Autodesk Fusion 360 part; units mm, degrees
(part 3 of 4)
  arc A160 (-35.8833, 38.7193) -> (-35.3833, 38.2193) centre (-35.3833, 38.7193) ccw
  line L159 (-35.8833, 38.7193) -> (-35.8833, 51.7193)
  arc A161 (-16.8333, -104.1557) -> (-16.3333, -104.6557) centre (-16.3333, -104.1557) ccw
  line L160 (-16.8333, -104.1557) -> (-16.8333, -91.1557)
  arc A162 (-16.3333, -90.6557) -> (-16.8333, -91.1557) centre (-16.3333, -91.1557) ccw
  line L161 (-16.3333, -90.6557) -> (-3.3333, -90.6557)
  arc A163 (-2.8333, -91.1557) -> (-3.3333, -90.6557) centre (-3.3333, -91.1557) ccw
  line L162 (-2.8333, -91.1557) -> (-2.8333, -104.1557)
  arc A164 (-3.3333, -104.6557) -> (-2.8333, -104.1557) centre (-3.3333, -104.1557) ccw
  line L163 (-3.3333, -104.6557) -> (-16.3333, -104.6557)
  line L164 (35.2668, 213.6443) -> (35.2667, 200.6443)
  arc A165 (34.7667, 200.1443) -> (35.2667, 200.6443) centre (34.7667, 200.6443) ccw
  line L165 (34.7667, 200.1443) -> (21.7667, 200.1443)
  arc A166 (21.2668, 200.6443) -> (21.7667, 200.1443) centre (21.7667, 200.6443) ccw
  line L166 (21.2668, 200.6443) -> (21.2667, 213.6443)
  arc A167 (21.7667, 214.1443) -> (21.2667, 213.6443) centre (21.7668, 213.6443) ccw
  line L167 (21.7667, 214.1443) -> (34.7667, 214.1443)
  arc A168 (35.2668, 213.6443) -> (34.7667, 214.1443) centre (34.7667, 213.6443) ccw
  arc A169 (-41.4333, -78.462) -> (-40.9333, -77.962) centre (-41.4333, -77.962) ccw
  line L168 (-41.4333, -78.462) -> (-54.4333, -78.462)
  arc A170 (-54.9333, -77.962) -> (-54.4333, -78.462) centre (-54.4333, -77.962) ccw
  line L169 (-54.9333, -77.962) -> (-54.9333, -64.962)
  arc A171 (-54.4333, -64.462) -> (-54.9333, -64.962) centre (-54.4333, -64.962) ccw
  line L170 (-54.4333, -64.462) -> (-41.4333, -64.462)
  arc A172 (-40.9333, -64.962) -> (-41.4333, -64.462) centre (-41.4333, -64.962) ccw
  line L171 (-40.9333, -64.962) -> (-40.9333, -77.962)
  line L172 (58.5792, -47.5057) -> (45.5792, -47.5057)
  arc A173 (45.0792, -47.0057) -> (45.5792, -47.5057) centre (45.5792, -47.0057) ccw
  line L173 (45.0792, -47.0057) -> (45.0792, -34.0057)
  arc A174 (45.5792, -33.5057) -> (45.0792, -34.0057) centre (45.5792, -34.0057) ccw
  line L174 (45.5792, -33.5057) -> (58.5792, -33.5057)
  arc A175 (59.0792, -34.0057) -> (58.5792, -33.5057) centre (58.5793, -34.0057) ccw
  line L175 (59.0792, -34.0057) -> (59.0793, -47.0057)
  arc A176 (58.5792, -47.5057) -> (59.0793, -47.0057) centre (58.5792, -47.0057) ccw
  line L176 (35.2667, -100.6807) -> (35.2667, -113.6807)
  arc A177 (34.7667, -114.1807) -> (35.2667, -113.6807) centre (34.7667, -113.6807) ccw
  line L177 (34.7667, -114.1807) -> (21.7667, -114.1807)
  arc A178 (21.2667, -113.6807) -> (21.7667, -114.1807) centre (21.7667, -113.6807) ccw
  line L178 (21.2667, -113.6807) -> (21.2667, -100.6807)
  arc A179 (21.7667, -100.1807) -> (21.2667, -100.6807) centre (21.7667, -100.6807) ccw
  line L179 (21.7667, -100.1807) -> (34.7667, -100.1807)
  arc A180 (35.2667, -100.6807) -> (34.7667, -100.1807) centre (34.7667, -100.6807) ccw
  line L180 (-41.4333, -126.087) -> (-54.4333, -126.087)
  arc A181 (-54.9333, -125.587) -> (-54.4333, -126.087) centre (-54.4333, -125.587) ccw
  line L181 (-54.9333, -125.587) -> (-54.9333, -112.587)
  arc A182 (-54.4333, -112.087) -> (-54.9333, -112.587) centre (-54.4333, -112.587) ccw
  line L182 (-54.4333, -112.087) -> (-41.4333, -112.087)
  arc A183 (-40.9333, -112.587) -> (-41.4333, -112.087) centre (-41.4333, -112.587) ccw
  line L183 (-40.9333, -112.587) -> (-40.9332, -125.587)
  arc A184 (-41.4333, -126.087) -> (-40.9332, -125.587) centre (-41.4333, -125.587) ccw
  line L184 (45.5792, -114.4682) -> (58.5792, -114.4682)
  arc A185 (59.0792, -114.9682) -> (58.5792, -114.4682) centre (58.5792, -114.9682) ccw
  line L185 (59.0792, -114.9682) -> (59.0792, -127.9682)
  arc A186 (58.5792, -128.4682) -> (59.0792, -127.9682) centre (58.5792, -127.9682) ccw
  line L186 (58.5792, -128.4682) -> (45.5792, -128.4682)
  arc A187 (45.0792, -127.9682) -> (45.5792, -128.4682) centre (45.5792, -127.9682) ccw
  line L187 (45.0792, -127.9682) -> (45.0792, -114.9682)
  arc A188 (45.5792, -114.4682) -> (45.0792, -114.9682) centre (45.5792, -114.9682) ccw
  arc A189 (15.7167, 33.4568) -> (16.2167, 33.9568) centre (15.7167, 33.9568) ccw
  line L188 (15.7167, 33.4568) -> (2.7167, 33.4568)
  arc A190 (2.2167, 33.9568) -> (2.7167, 33.4568) centre (2.7167, 33.9568) ccw
  line L189 (2.2167, 33.9568) -> (2.2167, 46.9568)
  arc A191 (2.7167, 47.4568) -> (2.2167, 46.9568) centre (2.7167, 46.9568) ccw
  line L190 (2.7167, 47.4568) -> (15.7167, 47.4568)
  arc A192 (16.2167, 46.9568) -> (15.7167, 47.4568) centre (15.7167, 46.9568) ccw
  line L191 (16.2167, 46.9568) -> (16.2167, 33.9568)
  arc A193 (-44.9083, 156.9943) -> (-45.4083, 156.4943) centre (-44.9082, 156.4943) ccw
  line L192 (-44.9083, 156.9943) -> (-31.9083, 156.9943)
  arc A194 (-31.4083, 156.4943) -> (-31.9083, 156.9943) centre (-31.9083, 156.4943) ccw
  line L193 (-31.4083, 156.4943) -> (-31.4083, 143.4943)
  arc A195 (-31.9083, 142.9943) -> (-31.4083, 143.4943) centre (-31.9083, 143.4943) ccw
  line L194 (-31.9083, 142.9943) -> (-44.9083, 142.9943)
  arc A196 (-45.4083, 143.4943) -> (-44.9083, 142.9943) centre (-44.9083, 143.4943) ccw
  line L195 (-45.4083, 143.4943) -> (-45.4083, 156.4943)
  arc A197 (45.0792, 91.1068) -> (45.5793, 90.6068) centre (45.5792, 91.1068) ccw
  line L196 (45.0792, 91.1068) -> (45.0792, 104.1068)
  arc A198 (45.5792, 104.6068) -> (45.0792, 104.1068) centre (45.5792, 104.1068) ccw
  line L197 (45.5792, 104.6068) -> (58.5792, 104.6068)
  arc A199 (59.0792, 104.1068) -> (58.5792, 104.6068) centre (58.5792, 104.1068) ccw
  line L198 (59.0792, 104.1068) -> (59.0792, 91.1068)
  arc A200 (58.5793, 90.6068) -> (59.0792, 91.1068) centre (58.5792, 91.1068) ccw
  line L199 (58.5793, 90.6068) -> (45.5793, 90.6068)
  line L200 (-46.8463, 155.4943) -> (-46.8463, 141.4943)
  arc A201 (-47.3463, 140.9943) -> (-46.8463, 141.4943) centre (-47.3463, 141.4943) ccw
  line L201 (-47.3463, 140.9943) -> (-53.3463, 140.9943)
  arc A202 (-53.8463, 141.4943) -> (-53.3463, 140.9943) centre (-53.3463, 141.4943) ccw
  line L202 (-53.8463, 141.4943) -> (-53.8462, 155.4943)
  arc A203 (-53.3463, 155.9943) -> (-53.8462, 155.4943) centre (-53.3463, 155.4943) ccw
  line L203 (-53.3463, 155.9943) -> (-47.3463, 155.9943)
  arc A204 (-46.8463, 155.4943) -> (-47.3463, 155.9943) centre (-47.3463, 155.4943) ccw
  line L204 (34.7667, 57.2693) -> (21.7667, 57.2693)
  arc A205 (21.2667, 57.7693) -> (21.7667, 57.2693) centre (21.7667, 57.7693) ccw
  line L205 (21.2667, 57.7693) -> (21.2667, 70.7693)
  arc A206 (21.7667, 71.2693) -> (21.2667, 70.7693) centre (21.7667, 70.7693) ccw
  line L206 (21.7667, 71.2693) -> (34.7667, 71.2693)
  arc A207 (35.2667, 70.7693) -> (34.7667, 71.2693) centre (34.7667, 70.7693) ccw
  line L207 (35.2667, 70.7693) -> (35.2667, 57.7693)
  arc A208 (34.7667, 57.2693) -> (35.2667, 57.7693) centre (34.7667, 57.7693) ccw
  line L208 (16.2167, -29.2432) -> (16.2167, -42.2432)
  arc A209 (15.7167, -42.7432) -> (16.2167, -42.2432) centre (15.7167, -42.2432) ccw
  line L209 (15.7167, -42.7432) -> (2.7167, -42.7432)
  arc A210 (2.2167, -42.2432) -> (2.7167, -42.7432) centre (2.7167, -42.2432) ccw
  line L210 (2.2167, -42.2432) -> (2.2167, -29.2432)
  arc A211 (2.7167, -28.7432) -> (2.2167, -29.2432) centre (2.7167, -29.2432) ccw
  line L211 (2.7167, -28.7432) -> (15.7167, -28.7432)
  arc A212 (16.2167, -29.2432) -> (15.7167, -28.7432) centre (15.7167, -29.2432) ccw
  line L212 (67.9431, 166.6443) -> (37.7667, 166.6443)
  line L213 (37.7667, 166.6443) -> (37.7668, 228.6)
  line L214 (37.7668, 228.6) -> (-61.7708, 228.6)
  line L215 (-61.7708, 228.6) -> (-61.7708, -231.4)
  line L216 (-61.7708, -231.4) -> (63.3431, -231.4)
  line L217 (63.3431, -231.4) -> (67.9431, -231.4)
  line L218 (67.9431, -231.4) -> (67.9431, 166.6443)
  line L219 (-2.8333, -53.0557) -> (-2.8333, -66.0557)
  arc A213 (-3.3333, -66.5557) -> (-2.8333, -66.0557) centre (-3.3333, -66.0557) ccw
  line L220 (-3.3333, -66.5557) -> (-16.3333, -66.5557)
  arc A214 (-16.8333, -66.0557) -> (-16.3333, -66.5557) centre (-16.3333, -66.0557) ccw
  line L221 (-16.8333, -66.0557) -> (-16.8333, -53.0557)
  arc A215 (-16.3333, -52.5557) -> (-16.8333, -53.0557) centre (-16.3333, -53.0557) ccw
  line L222 (-16.3333, -52.5557) -> (-3.3333, -52.5557)
  arc A216 (-2.8333, -53.0557) -> (-3.3333, -52.5557) centre (-3.3333, -53.0557) ccw
  line L223 (-37.8833, 120.8323) -> (-37.8833, 126.8323)
  arc A217 (-37.3833, 127.3323) -> (-37.8833, 126.8323) centre (-37.3833, 126.8323) ccw
  line L224 (-37.3833, 127.3323) -> (-23.3833, 127.3323)
  arc A218 (-22.8833, 126.8323) -> (-23.3833, 127.3323) centre (-23.3833, 126.8323) ccw
  line L225 (-22.8833, 126.8323) -> (-22.8833, 120.8323)
  arc A219 (-23.3833, 120.3323) -> (-22.8833, 120.8323) centre (-23.3833, 120.8323) ccw
  line L226 (-23.3833, 120.3323) -> (-37.3833, 120.3323)
  arc A220 (-37.8833, 120.8323) -> (-37.3833, 120.3323) centre (-37.3833, 120.8323) ccw
  arc A221 (2.7167, 85.5568) -> (2.2167, 85.0568) centre (2.7167, 85.0568) ccw
  line L227 (2.7167, 85.5568) -> (15.7167, 85.5568)
  arc A222 (16.2167, 85.0568) -> (15.7167, 85.5568) centre (15.7167, 85.0568) ccw
  line L228 (16.2167, 85.0568) -> (16.2167, 72.0568)
  arc A223 (15.7167, 71.5568) -> (16.2167, 72.0568) centre (15.7167, 72.0568) ccw
  line L229 (15.7167, 71.5568) -> (2.7167, 71.5568)
  arc A224 (2.2167, 72.0568) -> (2.7167, 71.5568) centre (2.7167, 72.0568) ccw
  line L230 (2.2167, 72.0568) -> (2.2167, 85.0568)
  arc A225 (15.7167, 162.0443) -> (16.2168, 162.5443) centre (15.7167, 162.5443) ccw
  line L231 (15.7167, 162.0443) -> (2.7168, 162.0443)
  arc A226 (2.2167, 162.5443) -> (2.7168, 162.0443) centre (2.7168, 162.5443) ccw
  line L232 (2.2167, 162.5443) -> (2.2168, 175.5443)
  arc A227 (2.7168, 176.0443) -> (2.2168, 175.5443) centre (2.7167, 175.5443) ccw
  line L233 (2.7168, 176.0443) -> (15.7167, 176.0443)
  arc A228 (16.2168, 175.5443) -> (15.7167, 176.0443) centre (15.7168, 175.5443) ccw
  line L234 (16.2168, 175.5443) -> (16.2168, 162.5443)
  line L235 (-22.9703, 155.4943) -> (-22.9703, 141.4943)
  arc A229 (-23.4703, 140.9943) -> (-22.9703, 141.4943) centre (-23.4703, 141.4943) ccw
  line L236 (-23.4703, 140.9943) -> (-29.4703, 140.9943)
  arc A230 (-29.9703, 141.4943) -> (-29.4703, 140.9943) centre (-29.4703, 141.4943) ccw
  line L237 (-29.9703, 141.4943) -> (-29.9703, 155.4943)
  arc A231 (-29.4703, 155.9943) -> (-29.9703, 155.4943) centre (-29.4702, 155.4943) ccw
  line L238 (-29.4703, 155.9943) -> (-23.4703, 155.9943)
  arc A232 (-22.9703, 155.4943) -> (-23.4703, 155.9943) centre (-23.4703, 155.4943) ccw
  line L239 (-16.3333, -33.5057) -> (-3.3333, -33.5057)
  arc A233 (-2.8333, -34.0057) -> (-3.3333, -33.5057) centre (-3.3333, -34.0057) ccw
  line L240 (-2.8333, -34.0057) -> (-2.8333, -47.0057)
  arc A234 (-3.3333, -47.5057) -> (-2.8333, -47.0057) centre (-3.3333, -47.0057) ccw
  line L241 (-3.3333, -47.5057) -> (-16.3333, -47.5057)
  arc A235 (-16.8333, -47.0057) -> (-16.3333, -47.5057) centre (-16.3333, -47.0057) ccw
  line L242 (-16.8333, -47.0057) -> (-16.8333, -34.0057)
  arc A236 (-16.3333, -33.5057) -> (-16.8333, -34.0057) centre (-16.3333, -34.0057) ccw
  line L243 (-21.8833, -181.6432) -> (-21.8833, -194.6432)
  arc A237 (-22.3833, -195.1432) -> (-21.8833, -194.6432) centre (-22.3833, -194.6432) ccw
  line L244 (-22.3833, -195.1432) -> (-35.3833, -195.1432)
  arc A238 (-35.8833, -194.6432) -> (-35.3833, -195.1432) centre (-35.3833, -194.6432) ccw
  line L245 (-35.8833, -194.6432) -> (-35.8833, -181.6432)
  arc A239 (-35.3833, -181.1432) -> (-35.8833, -181.6432) centre (-35.3833, -181.6432) ccw
  line L246 (-35.3833, -181.1432) -> (-22.3833, -181.1432)
  arc A240 (-21.8833, -181.6432) -> (-22.3833, -181.1432) centre (-22.3833, -181.6432) ccw
  arc A241 (2.7167, -9.6932) -> (2.2168, -10.1932) centre (2.7167, -10.1932) ccw
  line L247 (2.7167, -9.6932) -> (15.7167, -9.6932)
  arc A242 (16.2167, -10.1932) -> (15.7167, -9.6932) centre (15.7167, -10.1932) ccw
  line L248 (16.2167, -10.1932) -> (16.2167, -23.1932)
  arc A243 (15.7167, -23.6932) -> (16.2167, -23.1932) centre (15.7167, -23.1932) ccw
  line L249 (15.7167, -23.6932) -> (2.7167, -23.6932)
  arc A244 (2.2167, -23.1932) -> (2.7167, -23.6932) centre (2.7167, -23.1932) ccw
  line L250 (2.2167, -23.1932) -> (2.2168, -10.1932)
  line L251 (-54.9333, -101.7745) -> (-54.9333, -88.7745)
  arc A245 (-54.4333, -88.2745) -> (-54.9333, -88.7745) centre (-54.4333, -88.7745) ccw
  line L252 (-54.4333, -88.2745) -> (-41.4333, -88.2745)
  arc A246 (-40.9333, -88.7745) -> (-41.4333, -88.2745) centre (-41.4333, -88.7745) ccw
  line L253 (-40.9333, -88.7745) -> (-40.9333, -101.7745)
  arc A247 (-41.4333, -102.2745) -> (-40.9333, -101.7745) centre (-41.4333, -101.7745) ccw
  line L254 (-41.4333, -102.2745) -> (-54.4333, -102.2745)
  arc A248 (-54.9333, -101.7745) -> (-54.4333, -102.2745) centre (-54.4333, -101.7745) ccw
  circle A249 centre (42.9431, 161.6443) radius 1.5
  arc A250 (-21.8833, 32.6693) -> (-22.3833, 33.1693) centre (-22.3833, 32.6693) ccw
  line L255 (-21.8833, 32.6693) -> (-21.8833, 19.6693)
  arc A251 (-22.3833, 19.1693) -> (-21.8833, 19.6693) centre (-22.3833, 19.6693) ccw
  line L256 (-22.3833, 19.1693) -> (-35.3833, 19.1693)
  arc A252 (-35.8833, 19.6693) -> (-35.3833, 19.1693) centre (-35.3833, 19.6693) ccw
  line L257 (-35.8833, 19.6693) -> (-35.8833, 32.6693)
  arc A253 (-35.3833, 33.1693) -> (-35.8833, 32.6693) centre (-35.3833, 32.6693) ccw
  line L258 (-35.3833, 33.1693) -> (-22.3833, 33.1693)
  line L259 (35.2667, 32.6693) -> (35.2667, 19.6693)
  arc A254 (34.7667, 19.1693) -> (35.2667, 19.6693) centre (34.7667, 19.6693) ccw
  line L260 (34.7667, 19.1693) -> (21.7667, 19.1693)
  arc A255 (21.2667, 19.6693) -> (21.7667, 19.1693) centre (21.7667, 19.6693) ccw
  line L261 (21.2667, 19.6693) -> (21.2667, 32.6693)
  arc A256 (21.7667, 33.1693) -> (21.2667, 32.6693) centre (21.7667, 32.6693) ccw
  line L262 (21.7667, 33.1693) -> (34.7667, 33.1693)
  arc A257 (35.2667, 32.6693) -> (34.7667, 33.1693) centre (34.7667, 32.6693) ccw
  arc A258 (-2.8333, 123.1568) -> (-3.3333, 123.6568) centre (-3.3333, 123.1568) ccw
  line L263 (-2.8333, 123.1568) -> (-2.8333, 110.1568)
  arc A259 (-3.3333, 109.6568) -> (-2.8333, 110.1568) centre (-3.3333, 110.1568) ccw
  line L264 (-3.3333, 109.6568) -> (-16.3333, 109.6568)
  arc A260 (-16.8333, 110.1568) -> (-16.3333, 109.6568) centre (-16.3333, 110.1568) ccw
  line L265 (-16.8333, 110.1568) -> (-16.8333, 123.1568)
  arc A261 (-16.3333, 123.6568) -> (-16.8333, 123.1568) centre (-16.3333, 123.1568) ccw
  line L266 (-16.3333, 123.6568) -> (-3.3333, 123.6568)
  line L267 (35.2667, 89.8193) -> (35.2667, 76.8193)
  arc A262 (34.7667, 76.3193) -> (35.2667, 76.8193) centre (34.7667, 76.8193) ccw
  line L268 (34.7667, 76.3193) -> (21.7667, 76.3193)
  arc A263 (21.2667, 76.8193) -> (21.7667, 76.3193) centre (21.7667, 76.8193) ccw
  line L269 (21.2667, 76.8193) -> (21.2667, 89.8193)
  arc A264 (21.7667, 90.3193) -> (21.2667, 89.8193) centre (21.7667, 89.8193) ccw
  line L270 (21.7667, 90.3193) -> (34.7667, 90.3193)
  arc A265 (35.2667, 89.8193) -> (34.7667, 90.3193) centre (34.7667, 89.8193) ccw
  line L271 (-35.3833, -62.0807) -> (-22.3833, -62.0807)
  arc A266 (-21.8833, -62.5807) -> (-22.3833, -62.0807) centre (-22.3833, -62.5807) ccw
  line L272 (-21.8833, -62.5807) -> (-21.8833, -75.5807)
  arc A267 (-22.3833, -76.0807) -> (-21.8833, -75.5807) centre (-22.3833, -75.5807) ccw
  line L273 (-22.3833, -76.0807) -> (-35.3833, -76.0807)
  arc A268 (-35.8833, -75.5807) -> (-35.3833, -76.0807) centre (-35.3833, -75.5807) ccw
  line L274 (-35.8833, -75.5807) -> (-35.8833, -62.5807)
  arc A269 (-35.3833, -62.0807) -> (-35.8833, -62.5807) centre (-35.3833, -62.5807) ccw
  arc A270 (21.7667, -23.9807) -> (21.2667, -24.4807) centre (21.7667, -24.4807) ccw
  line L275 (21.7667, -23.9807) -> (34.7667, -23.9807)
  arc A271 (35.2667, -24.4807) -> (34.7667, -23.9807) centre (34.7667, -24.4807) ccw
  line L276 (35.2667, -24.4807) -> (35.2667, -37.4807)
  arc A272 (34.7667, -37.9807) -> (35.2667, -37.4807) centre (34.7667, -37.4807) ccw
  line L277 (34.7667, -37.9807) -> (21.7667, -37.9807)
  arc A273 (21.2667, -37.4807) -> (21.7667, -37.9807) centre (21.7667, -37.4807) ccw
  line L278 (21.2667, -37.4807) -> (21.2667, -24.4807)
  line L279 (-40.9333, -162.5932) -> (-40.9333, -175.5932)
  arc A274 (-41.4333, -176.0932) -> (-40.9333, -175.5932) centre (-41.4333, -175.5932) ccw
  line L280 (-41.4333, -176.0932) -> (-54.4333, -176.0932)
  arc A275 (-54.9333, -175.5932) -> (-54.4333, -176.0932) centre (-54.4333, -175.5932) ccw
  line L281 (-54.9333, -175.5932) -> (-54.9333, -162.5932)
  arc A276 (-54.4333, -162.0932) -> (-54.9333, -162.5932) centre (-54.4333, -162.5932) ccw
  line L282 (-54.4333, -162.0932) -> (-41.4333, -162.0932)
  arc A277 (-40.9333, -162.5932) -> (-41.4333, -162.0932) centre (-41.4333, -162.5932) ccw
  arc A278 (58.5792, -71.3182) -> (59.0793, -70.8182) centre (58.5792, -70.8182) ccw
  line L283 (58.5792, -71.3182) -> (45.5792, -71.3182)
  arc A279 (45.0792, -70.8182) -> (45.5792, -71.3182) centre (45.5792, -70.8182) ccw
  line L284 (45.0792, -70.8182) -> (45.0792, -57.8182)
  arc A280 (45.5792, -57.3182) -> (45.0792, -57.8182) centre (45.5792, -57.8182) ccw
  line L285 (45.5792, -57.3182) -> (58.5792, -57.3182)
  arc A281 (59.0792, -57.8182) -> (58.5792, -57.3182) centre (58.5792, -57.8182) ccw
  line L286 (59.0792, -57.8182) -> (59.0793, -70.8182)
  line L287 (16.2167, 194.5943) -> (16.2168, 181.5943)
  arc A282 (15.7167, 181.0943) -> (16.2168, 181.5943) centre (15.7167, 181.5943) ccw
  line L288 (15.7167, 181.0943) -> (2.7168, 181.0943)
  arc A283 (2.2168, 181.5943) -> (2.7168, 181.0943) centre (2.7167, 181.5943) ccw
  line L289 (2.2168, 181.5943) -> (2.2167, 194.5943)
  arc A284 (2.7168, 195.0943) -> (2.2167, 194.5943) centre (2.7167, 194.5943) ccw
  line L290 (2.7168, 195.0943) -> (15.7168, 195.0943)
  arc A285 (16.2167, 194.5943) -> (15.7168, 195.0943) centre (15.7167, 194.5943) ccw
  arc A286 (-35.8833, 105.3943) -> (-35.3833, 104.8943) centre (-35.3833, 105.3943) ccw
  line L291 (-35.8833, 105.3943) -> (-35.8833, 118.3943)
  arc A287 (-35.3833, 118.8943) -> (-35.8833, 118.3943) centre (-35.3833, 118.3943) ccw
  line L292 (-35.3833, 118.8943) -> (-22.3833, 118.8943)
  arc A288 (-21.8833, 118.3943) -> (-22.3833, 118.8943) centre (-22.3833, 118.3943) ccw
  line L293 (-21.8833, 118.3943) -> (-21.8833, 105.3943)
  arc A289 (-22.3833, 104.8943) -> (-21.8833, 105.3943) centre (-22.3833, 105.3943) ccw
  line L294 (-22.3833, 104.8943) -> (-35.3833, 104.8943)
  line L295 (-41.4333, 190.6193) -> (-54.4333, 190.6193)
  arc A290 (-54.9332, 191.1193) -> (-54.4333, 190.6193) centre (-54.4333, 191.1193) ccw
  line L296 (-54.9332, 191.1193) -> (-54.9332, 204.1193)
  arc A291 (-54.4332, 204.6193) -> (-54.9332, 204.1193) centre (-54.4333, 204.1193) ccw
  line L297 (-54.4332, 204.6193) -> (-41.4333, 204.6193)
  arc A292 (-40.9332, 204.1193) -> (-41.4333, 204.6193) centre (-41.4332, 204.1193) ccw
  line L298 (-40.9332, 204.1193) -> (-40.9333, 191.1193)
  arc A293 (-41.4333, 190.6193) -> (-40.9333, 191.1193) centre (-41.4333, 191.1193) ccw
  arc A294 (-16.8333, -85.1057) -> (-16.3333, -85.6057) centre (-16.3333, -85.1057) ccw
  line L299 (-16.8333, -85.1057) -> (-16.8333, -72.1057)
  arc A295 (-16.3333, -71.6057) -> (-16.8333, -72.1057) centre (-16.3333, -72.1057) ccw
  line L300 (-16.3333, -71.6057) -> (-3.3333, -71.6057)
  arc A296 (-2.8333, -72.1057) -> (-3.3333, -71.6057) centre (-3.3333, -72.1057) ccw
  line L301 (-2.8333, -72.1057) -> (-2.8333, -85.1057)
  arc A297 (-3.3333, -85.6057) -> (-2.8333, -85.1057) centre (-3.3333, -85.1057) ccw
  line L302 (-3.3333, -85.6057) -> (-16.3333, -85.6057)
  line L303 (-35.3833, 195.0943) -> (-22.3833, 195.0943)
  arc A298 (-21.8833, 194.5943) -> (-22.3833, 195.0943) centre (-22.3832, 194.5943) ccw
  line L304 (-21.8833, 194.5943) -> (-21.8833, 181.5943)
  arc A299 (-22.3833, 181.0943) -> (-21.8833, 181.5943) centre (-22.3833, 181.5943) ccw
  line L305 (-22.3833, 181.0943) -> (-35.3833, 181.0943)
  arc A300 (-35.8833, 181.5943) -> (-35.3833, 181.0943) centre (-35.3833, 181.5943) ccw
  line L306 (-35.8833, 181.5943) -> (-35.8833, 194.5943)
  arc A301 (-35.3833, 195.0943) -> (-35.8833, 194.5943) centre (-35.3833, 194.5943) ccw
  line L307 (15.7167, 14.4068) -> (2.7167, 14.4068)
  arc A302 (2.2167, 14.9068) -> (2.7167, 14.4068) centre (2.7167, 14.9068) ccw
  line L308 (2.2167, 14.9068) -> (2.2167, 27.9068)
  arc A303 (2.7167, 28.4068) -> (2.2167, 27.9068) centre (2.7167, 27.9068) ccw
  line L309 (2.7167, 28.4068) -> (15.7167, 28.4068)
  arc A304 (16.2167, 27.9068) -> (15.7167, 28.4068) centre (15.7167, 27.9068) ccw
  line L310 (16.2167, 27.9068) -> (16.2167, 14.9068)
  arc A305 (15.7167, 14.4068) -> (16.2167, 14.9068) centre (15.7167, 14.9068) ccw
  line L311 (-16.8333, 10.1443) -> (-16.8333, 23.1443)
  arc A306 (-16.3333, 23.6443) -> (-16.8333, 23.1443) centre (-16.3333, 23.1443) ccw
  line L312 (-16.3333, 23.6443) -> (-3.3333, 23.6443)
  arc A307 (-2.8333, 23.1443) -> (-3.3333, 23.6443) centre (-3.3333, 23.1443) ccw
  line L313 (-2.8333, 23.1443) -> (-2.8333, 10.1443)
  arc A308 (-3.3333, 9.6443) -> (-2.8333, 10.1443) centre (-3.3333, 10.1443) ccw
  line L314 (-3.3333, 9.6443) -> (-16.3333, 9.6443)
  arc A309 (-16.8333, 10.1443) -> (-16.3333, 9.6443) centre (-16.3333, 10.1443) ccw
  line L315 (25.2417, -195.1432) -> (12.2417, -195.1432)
  arc A310 (11.7417, -194.6432) -> (12.2417, -195.1432) centre (12.2417, -194.6432) ccw
  line L316 (11.7417, -194.6432) -> (11.7417, -181.6432)
  arc A311 (12.2417, -181.1432) -> (11.7417, -181.6432) centre (12.2417, -181.6432) ccw
  line L317 (12.2417, -181.1432) -> (25.2417, -181.1432)
  arc A312 (25.7417, -181.6432) -> (25.2417, -181.1432) centre (25.2417, -181.6432) ccw
  line L318 (25.7417, -181.6432) -> (25.7417, -194.6432)
  arc A313 (25.2417, -195.1432) -> (25.7417, -194.6432) centre (25.2417, -194.6432) ccw
  arc A314 (-40.9333, 125.538) -> (-41.4333, 126.038) centre (-41.4333, 125.538) ccw
  line L319 (-40.9333, 125.538) -> (-40.9333, 112.538)
  arc A315 (-41.4333, 112.038) -> (-40.9333, 112.538) centre (-41.4333, 112.538) ccw
  line L320 (-41.4333, 112.038) -> (-54.4333, 112.038)
  arc A316 (-54.9333, 112.538) -> (-54.4333, 112.038) centre (-54.4333, 112.538) ccw
  line L321 (-54.9333, 112.538) -> (-54.9333, 125.538)
  arc A317 (-54.4333, 126.038) -> (-54.9333, 125.538) centre (-54.4333, 125.538) ccw
  line L322 (-54.4333, 126.038) -> (-41.4333, 126.038)
  arc A318 (-37.3833, 103.4563) -> (-37.8833, 102.9563) centre (-37.3833, 102.9563) ccw
  line L323 (-37.3833, 103.4563) -> (-23.3833, 103.4563)
  arc A319 (-22.8833, 102.9563) -> (-23.3833, 103.4563) centre (-23.3833, 102.9563) ccw
  line L324 (-22.8833, 102.9563) -> (-22.8833, 96.9563)
  arc A320 (-23.3833, 96.4563) -> (-22.8833, 96.9563) centre (-23.3833, 96.9563) ccw
  line L325 (-23.3833, 96.4563) -> (-37.3833, 96.4563)
  arc A321 (-37.8833, 96.9563) -> (-37.3833, 96.4563) centre (-37.3833, 96.9563) ccw
  line L326 (-37.8833, 96.9563) -> (-37.8833, 102.9563)
  arc A322 (6.6917, -162.5932) -> (6.1917, -162.0932) centre (6.1917, -162.5932) ccw
  line L327 (6.6917, -162.5932) -> (6.6917, -175.5932)
  arc A323 (6.1917, -176.0932) -> (6.6917, -175.5932) centre (6.1917, -175.5932) ccw
  line L328 (6.1917, -176.0932) -> (-6.8083, -176.0932)
  arc A324 (-7.3083, -175.5932) -> (-6.8083, -176.0932) centre (-6.8083, -175.5932) ccw
  line L329 (-7.3083, -175.5932) -> (-7.3083, -162.5932)
  arc A325 (-6.8083, -162.0932) -> (-7.3083, -162.5932) centre (-6.8083, -162.5932) ccw
  line L330 (-6.8083, -162.0932) -> (6.1917, -162.0932)
  arc A326 (15.7167, -118.9432) -> (16.2167, -118.4432) centre (15.7167, -118.4432) ccw
  line L331 (15.7167, -118.9432) -> (2.7167, -118.9432)
  arc A327 (2.2167, -118.4432) -> (2.7167, -118.9432) centre (2.7167, -118.4432) ccw
  line L332 (2.2167, -118.4432) -> (2.2167, -105.4432)
  arc A328 (2.7167, -104.9432) -> (2.2167, -105.4432) centre (2.7167, -105.4432) ccw
  line L333 (2.7167, -104.9432) -> (15.7167, -104.9432)
  arc A329 (16.2167, -105.4432) -> (15.7167, -104.9432) centre (15.7167, -105.4432) ccw
  line L334 (16.2167, -105.4432) -> (16.2167, -118.4432)
  line L335 (-3.3333, 85.8443) -> (-16.3333, 85.8443)
  arc A330 (-16.8333, 86.3443) -> (-16.3333, 85.8443) centre (-16.3333, 86.3443) ccw
  line L336 (-16.8333, 86.3443) -> (-16.8333, 99.3443)
  arc A331 (-16.3333, 99.8443) -> (-16.8333, 99.3443) centre (-16.3333, 99.3443) ccw
  line L337 (-16.3333, 99.8443) -> (-3.3333, 99.8443)
  arc A332 (-2.8333, 99.3443) -> (-3.3333, 99.8443) centre (-3.3333, 99.3443) ccw
  line L338 (-2.8333, 99.3443) -> (-2.8332, 86.3443)
  arc A333 (-3.3333, 85.8443) -> (-2.8332, 86.3443) centre (-3.3333, 86.3443) ccw
  line L339 (-3.3333, 47.7443) -> (-16.3333, 47.7443)
  arc A334 (-16.8333, 48.2443) -> (-16.3333, 47.7443) centre (-16.3333, 48.2443) ccw
  line L340 (-16.8333, 48.2443) -> (-16.8333, 61.2443)
  arc A335 (-16.3333, 61.7443) -> (-16.8333, 61.2443) centre (-16.3333, 61.2443) ccw
  line L341 (-16.3333, 61.7443) -> (-3.3333, 61.7443)
  arc A336 (-2.8333, 61.2443) -> (-3.3333, 61.7443) centre (-3.3333, 61.2443) ccw
  line L342 (-2.8333, 61.2443) -> (-2.8333, 48.2443)
  arc A337 (-3.3333, 47.7443) -> (-2.8333, 48.2443) centre (-3.3333, 48.2443) ccw
  line L343 (35.2667, -127.3495) -> (35.2667, -140.3495)
  arc A338 (34.7667, -140.8495) -> (35.2667, -140.3495) centre (34.7667, -140.3495) ccw
  line L344 (34.7667, -140.8495) -> (21.7667, -140.8495)
  arc A339 (21.2667, -140.3495) -> (21.7667, -140.8495) centre (21.7667, -140.3495) ccw
  line L345 (21.2667, -140.3495) -> (21.2667, -127.3495)
  arc A340 (21.7667, -126.8495) -> (21.2667, -127.3495) centre (21.7667, -127.3495) ccw
  line L346 (21.7667, -126.8495) -> (34.7667, -126.8495)
  arc A341 (35.2667, -127.3495) -> (34.7667, -126.8495) centre (34.7667, -127.3495) ccw
  arc A342 (58.5792, -109.4182) -> (59.0792, -108.9182) centre (58.5792, -108.9182) ccw
  line L347 (58.5792, -109.4182) -> (45.5792, -109.4182)
  arc A343 (45.0792, -108.9182) -> (45.5792, -109.4182) centre (45.5792, -108.9182) ccw
  line L348 (45.0792, -108.9182) -> (45.0792, -95.9182)
  arc A344 (45.5792, -95.4182) -> (45.0792, -95.9182) centre (45.5792, -95.9182) ccw
  line L349 (45.5792, -95.4182) -> (58.5792, -95.4182)
  arc A345 (59.0792, -95.9182) -> (58.5792, -95.4182) centre (58.5792, -95.9182) ccw
  line L350 (59.0792, -95.9182) -> (59.0792, -108.9182)
  line L351 (-35.3833, -81.1307) -> (-22.3833, -81.1307)
  arc A346 (-21.8833, -81.6307) -> (-22.3833, -81.1307) centre (-22.3833, -81.6307) ccw
  line L352 (-21.8833, -81.6307) -> (-21.8833, -94.6307)
  arc A347 (-22.3833, -95.1307) -> (-21.8833, -94.6307) centre (-22.3833, -94.6307) ccw
  line L353 (-22.3833, -95.1307) -> (-35.3833, -95.1307)
  arc A348 (-35.8833, -94.6307) -> (-35.3833, -95.1307) centre (-35.3833, -94.6307) ccw
  line L354 (-35.8833, -94.6307) -> (-35.8833, -81.6307)
  arc A349 (-35.3833, -81.1307) -> (-35.8833, -81.6307) centre (-35.3833, -81.6307) ccw
  arc A350 (15.7167, 90.6068) -> (16.2167, 91.1068) centre (15.7167, 91.1068) ccw
  line L355 (15.7167, 90.6068) -> (2.7167, 90.6068)
  arc A351 (2.2167, 91.1068) -> (2.7167, 90.6068) centre (2.7167, 91.1068) ccw
  line L356 (2.2167, 91.1068) -> (2.2167, 104.1068)
  arc A352 (2.7167, 104.6068) -> (2.2167, 104.1068) centre (2.7167, 104.1068) ccw
  line L357 (2.7167, 104.6068) -> (15.7167, 104.6068)
  arc A353 (16.2167, 104.1068) -> (15.7167, 104.6068) centre (15.7167, 104.1068) ccw
  line L358 (16.2167, 104.1068) -> (16.2167, 91.1068)
  line L359 (45.5792, -14.4557) -> (58.5792, -14.4557)
  arc A354 (59.0792, -14.9557) -> (58.5792, -14.4557) centre (58.5792, -14.9557) ccw
  line L360 (59.0792, -14.9557) -> (59.0792, -27.9557)
  arc A355 (58.5792, -28.4557) -> (59.0792, -27.9557) centre (58.5792, -27.9557) ccw
  line L361 (58.5792, -28.4557) -> (45.5792, -28.4557)
  arc A356 (45.0792, -27.9557) -> (45.5792, -28.4557) centre (45.5792, -27.9557) ccw
  line L362 (45.0792, -27.9557) -> (45.0792, -14.9557)
  arc A357 (45.5792, -14.4557) -> (45.0792, -14.9557) centre (45.5792, -14.9557) ccw
  arc A358 (34.7667, 0.1193) -> (35.2667, 0.6193) centre (34.7667, 0.6193) ccw
  line L363 (34.7667, 0.1193) -> (21.7667, 0.1193)
  arc A359 (21.2667, 0.6193) -> (21.7667, 0.1193) centre (21.7667, 0.6193) ccw
  line L364 (21.2667, 0.6193) -> (21.2667, 13.6193)
  arc A360 (21.7667, 14.1193) -> (21.2667, 13.6193) centre (21.7667, 13.6193) ccw
  line L365 (21.7667, 14.1193) -> (34.7667, 14.1193)
  arc A361 (35.2667, 13.6193) -> (34.7667, 14.1193) centre (34.7667, 13.6193) ccw
  line L366 (35.2667, 13.6193) -> (35.2667, 0.6193)
  arc A362 (45.5792, 66.5068) -> (45.0793, 66.0068) centre (45.5792, 66.0068) ccw
  line L367 (45.5792, 66.5068) -> (58.5792, 66.5068)
  arc A363 (59.0792, 66.0068) -> (58.5792, 66.5068) centre (58.5792, 66.0068) ccw
  line L368 (59.0792, 66.0068) -> (59.0793, 53.0068)
  arc A364 (58.5792, 52.5068) -> (59.0793, 53.0068) centre (58.5792, 53.0068) ccw
  line L369 (58.5792, 52.5068) -> (45.5792, 52.5068)
  arc A365 (45.0792, 53.0068) -> (45.5792, 52.5068) centre (45.5792, 53.0068) ccw
  line L370 (45.0792, 53.0068) -> (45.0793, 66.0068)
  arc A366 (-9.2463, -147.137) -> (-8.7463, -146.637) centre (-9.2463, -146.637) ccw
  line L371 (-9.2463, -147.137) -> (-15.2463, -147.137)
  arc A367 (-15.7463, -146.637) -> (-15.2463, -147.137) centre (-15.2463, -146.637) ccw
  line L372 (-15.7463, -146.637) -> (-15.7463, -132.637)
  arc A368 (-15.2463, -132.137) -> (-15.7463, -132.637) centre (-15.2463, -132.637) ccw
  line L373 (-15.2463, -132.137) -> (-9.2463, -132.137)
  arc A369 (-8.7463, -132.637) -> (-9.2463, -132.137) centre (-9.2463, -132.637) ccw
  line L374 (-8.7463, -132.637) -> (-8.7463, -146.637)
  line L375 (25.2417, -214.1932) -> (12.2417, -214.1932)
  arc A370 (11.7417, -213.6932) -> (12.2417, -214.1932) centre (12.2417, -213.6932) ccw
  line L376 (11.7417, -213.6932) -> (11.7417, -200.6932)
  arc A371 (12.2417, -200.1932) -> (11.7417, -200.6932) centre (12.2417, -200.6932) ccw
  line L377 (12.2417, -200.1932) -> (25.2417, -200.1932)
  arc A372 (25.7417, -200.6932) -> (25.2417, -200.1932) centre (25.2417, -200.6932) ccw
  line L378 (25.7417, -200.6932) -> (25.7417, -213.6932)
  arc A373 (25.2417, -214.1932) -> (25.7417, -213.6932) centre (25.2417, -213.6932) ccw
  line L379 (-15.7463, 141.4943) -> (-15.7463, 155.4943)
  arc A374 (-15.2463, 155.9943) -> (-15.7463, 155.4943) centre (-15.2463, 155.4943) ccw
  line L380 (-15.2463, 155.9943) -> (-9.2463, 155.9943)
  arc A375 (-8.7463, 155.4943) -> (-9.2463, 155.9943) centre (-9.2462, 155.4943) ccw
  line L381 (-8.7463, 155.4943) -> (-8.7463, 141.4943)
  arc A376 (-9.2463, 140.9943) -> (-8.7463, 141.4943) centre (-9.2463, 141.4943) ccw
  line L382 (-9.2463, 140.9943) -> (-15.2463, 140.9943)
  arc A377 (-15.7463, 141.4943) -> (-15.2463, 140.9943) centre (-15.2463, 141.4943) ccw
  line L383 (2.7167, -85.8932) -> (15.7167, -85.8932)
  arc A378 (16.2167, -86.3932) -> (15.7167, -85.8932) centre (15.7167, -86.3932) ccw
  line L384 (16.2167, -86.3932) -> (16.2167, -99.3932)
  arc A379 (15.7167, -99.8932) -> (16.2167, -99.3932) centre (15.7167, -99.3932) ccw
  line L385 (15.7167, -99.8932) -> (2.7167, -99.8932)
  arc A380 (2.2167, -99.3932) -> (2.7167, -99.8932) centre (2.7167, -99.3932) ccw
  line L386 (2.2167, -99.3932) -> (2.2167, -86.3932)
  arc A381 (2.7167, -85.8932) -> (2.2167, -86.3932) centre (2.7167, -86.3932) ccw
  arc A382 (-22.3833, -130.8495) -> (-21.8833, -130.3495) centre (-22.3833, -130.3495) ccw
  line L387 (-22.3833, -130.8495) -> (-35.3833, -130.8495)
  arc A383 (-35.8833, -130.3495) -> (-35.3833, -130.8495) centre (-35.3833, -130.3495) ccw
  line L388 (-35.8833, -130.3495) -> (-35.8833, -117.3495)
  arc A384 (-35.3833, -116.8495) -> (-35.8833, -117.3495) centre (-35.3833, -117.3495) ccw
  line L389 (-35.3833, -116.8495) -> (-22.3833, -116.8495)
  arc A385 (-21.8833, -117.3495) -> (-22.3833, -116.8495) centre (-22.3833, -117.3495) ccw
  line L390 (-21.8833, -117.3495) -> (-21.8833, -130.3495)
  arc A386 (-54.4333, 102.2255) -> (-54.9333, 101.7255) centre (-54.4333, 101.7255) ccw
  line L391 (-54.4333, 102.2255) -> (-41.4333, 102.2255)
  arc A387 (-40.9333, 101.7255) -> (-41.4333, 102.2255) centre (-41.4333, 101.7255) ccw
  line L392 (-40.9333, 101.7255) -> (-40.9333, 88.7255)
  arc A388 (-41.4333, 88.2255) -> (-40.9333, 88.7255) centre (-41.4333, 88.7255) ccw
  line L393 (-41.4333, 88.2255) -> (-54.4333, 88.2255)
  arc A389 (-54.9333, 88.7255) -> (-54.4333, 88.2255) centre (-54.4333, 88.7255) ccw
  line L394 (-54.9333, 88.7255) -> (-54.9333, 101.7255)
  line L395 (-34.3833, -132.2875) -> (-20.3833, -132.2875)
  arc A390 (-19.8833, -132.7875) -> (-20.3833, -132.2875) centre (-20.3833, -132.7875) ccw
  line L396 (-19.8833, -132.7875) -> (-19.8833, -138.7875)
  arc A391 (-20.3833, -139.2875) -> (-19.8833, -138.7875) centre (-20.3833, -138.7875) ccw
  line L397 (-20.3833, -139.2875) -> (-34.3833, -139.2875)
  arc A392 (-34.8833, -138.7875) -> (-34.3833, -139.2875) centre (-34.3833, -138.7875) ccw
  line L398 (-34.8833, -138.7875) -> (-34.8833, -132.7875)
  arc A393 (-34.3833, -132.2875) -> (-34.8833, -132.7875) centre (-34.3833, -132.7875) ccw
  arc A394 (8.1297, 141.4943) -> (8.6297, 140.9943) centre (8.6298, 141.4943) ccw
  line L399 (8.1297, 141.4943) -> (8.1297, 155.4943)
  arc A395 (8.6297, 155.9943) -> (8.1297, 155.4943) centre (8.6297, 155.4943) ccw
  line L400 (8.6297, 155.9943) -> (14.6298, 155.9943)
  arc A396 (15.1297, 155.4943) -> (14.6298, 155.9943) centre (14.6297, 155.4943) ccw
  line L401 (15.1297, 155.4943) -> (15.1297, 141.4943)
  arc A397 (14.6298, 140.9943) -> (15.1297, 141.4943) centre (14.6297, 141.4943) ccw
  line L402 (14.6298, 140.9943) -> (8.6297, 140.9943)
  line L403 (58.5792, 9.6443) -> (45.5792, 9.6443)
  arc A398 (45.0792, 10.1443) -> (45.5792, 9.6443) centre (45.5792, 10.1443) ccw
  line L404 (45.0792, 10.1443) -> (45.0793, 23.1443)
  arc A399 (45.5792, 23.6443) -> (45.0793, 23.1443) centre (45.5792, 23.1443) ccw
  line L405 (45.5792, 23.6443) -> (58.5792, 23.6443)
  arc A400 (59.0792, 23.1443) -> (58.5792, 23.6443) centre (58.5792, 23.1443) ccw
  line L406 (59.0792, 23.1443) -> (59.0793, 10.1443)
  arc A401 (58.5792, 9.6443) -> (59.0793, 10.1443) centre (58.5792, 10.1443) ccw
  line L407 (59.0792, 46.9568) -> (59.0793, 33.9568)
  arc A402 (58.5792, 33.4568) -> (59.0793, 33.9568) centre (58.5792, 33.9568) ccw
  line L408 (58.5792, 33.4568) -> (45.5792, 33.4568)
  arc A403 (45.0792, 33.9568) -> (45.5792, 33.4568) centre (45.5792, 33.9568) ccw
  line L409 (45.0792, 33.9568) -> (45.0792, 46.9568)
  arc A404 (45.5792, 47.4568) -> (45.0792, 46.9568) centre (45.5792, 46.9568) ccw
  line L410 (45.5792, 47.4568) -> (58.5792, 47.4568)
  arc A405 (59.0792, 46.9568) -> (58.5792, 47.4568) centre (58.5792, 46.9568) ccw
  line L411 (-53.9333, -53.0245) -> (-53.9333, -47.0245)
  arc A406 (-53.4333, -46.5245) -> (-53.9333, -47.0245) centre (-53.4333, -47.0245) ccw
  line L412 (-53.4333, -46.5245) -> (-39.4333, -46.5245)
  arc A407 (-38.9333, -47.0245) -> (-39.4333, -46.5245) centre (-39.4333, -47.0245) ccw
  line L413 (-38.9333, -47.0245) -> (-38.9333, -53.0245)
  arc A408 (-39.4333, -53.5245) -> (-38.9333, -53.0245) centre (-39.4333, -53.0245) ccw
  line L414 (-39.4333, -53.5245) -> (-53.4333, -53.5245)
  arc A409 (-53.9333, -53.0245) -> (-53.4333, -53.5245) centre (-53.4333, -53.0245) ccw
  line L415 (-2.8333, 4.0943) -> (-2.8333, -8.9057)
  arc A410 (-3.3333, -9.4057) -> (-2.8333, -8.9057) centre (-3.3333, -8.9057) ccw
  line L416 (-3.3333, -9.4057) -> (-16.3333, -9.4057)
  arc A411 (-16.8333, -8.9057) -> (-16.3333, -9.4057) centre (-16.3333, -8.9057) ccw
  line L417 (-16.8333, -8.9057) -> (-16.8333, 4.0943)
  arc A412 (-16.3333, 4.5943) -> (-16.8333, 4.0943) centre (-16.3333, 4.0943) ccw
  line L418 (-16.3333, 4.5943) -> (-3.3333, 4.5943)
  arc A413 (-2.8333, 4.0943) -> (-3.3333, 4.5943) centre (-3.3333, 4.0943) ccw
  line L419 (45.5792, 85.5568) -> (58.5792, 85.5568)
  arc A414 (59.0792, 85.0568) -> (58.5792, 85.5568) centre (58.5792, 85.0568) ccw
  line L420 (59.0792, 85.0568) -> (59.0792, 72.0568)
  arc A415 (58.5792, 71.5568) -> (59.0792, 72.0568) centre (58.5792, 72.0568) ccw
  line L421 (58.5792, 71.5568) -> (45.5792, 71.5568)
  arc A416 (45.0792, 72.0568) -> (45.5792, 71.5568) centre (45.5792, 72.0568) ccw
  line L422 (45.0792, 72.0568) -> (45.0792, 85.0568)
  arc A417 (45.5792, 85.5568) -> (45.0792, 85.0568) centre (45.5792, 85.0568) ccw
  arc A418 (-21.8833, -24.4807) -> (-22.3833, -23.9807) centre (-22.3833, -24.4807) ccw
  line L423 (-21.8833, -24.4807) -> (-21.8833, -37.4807)
  arc A419 (-22.3833, -37.9807) -> (-21.8833, -37.4807) centre (-22.3833, -37.4807) ccw
  line L424 (-22.3833, -37.9807) -> (-35.3833, -37.9807)
  arc A420 (-35.8833, -37.4807) -> (-35.3833, -37.9807) centre (-35.3833, -37.4807) ccw
  line L425 (-35.8833, -37.4807) -> (-35.8833, -24.4807)
  arc A421 (-35.3833, -23.9807) -> (-35.8833, -24.4807) centre (-35.3833, -24.4807) ccw
  line L426 (-35.3833, -23.9807) -> (-22.3833, -23.9807)
  line L427 (-54.4333, 78.413) -> (-41.4333, 78.413)
  arc A422 (-40.9333, 77.913) -> (-41.4333, 78.413) centre (-41.4333, 77.913) ccw
  line L428 (-40.9333, 77.913) -> (-40.9333, 64.913)
  arc A423 (-41.4333, 64.413) -> (-40.9333, 64.913) centre (-41.4333, 64.913) ccw
  line L429 (-41.4333, 64.413) -> (-54.4333, 64.413)
  arc A424 (-54.9333, 64.913) -> (-54.4333, 64.413) centre (-54.4333, 64.913) ccw
  line L430 (-54.9333, 64.913) -> (-54.9333, 77.913)
  arc A425 (-54.4333, 78.413) -> (-54.9333, 77.913) centre (-54.4333, 77.913) ccw
  arc A426 (15.7167, -61.7932) -> (16.2167, -61.2932) centre (15.7167, -61.2932) ccw
  line L431 (15.7167, -61.7932) -> (2.7167, -61.7932)
  arc A427 (2.2167, -61.2932) -> (2.7167, -61.7932) centre (2.7167, -61.2932) ccw
  line L432 (2.2167, -61.2932) -> (2.2167, -48.2932)
  arc A428 (2.7167, -47.7932) -> (2.2167, -48.2932) centre (2.7167, -48.2932) ccw
  line L433 (2.7167, -47.7932) -> (15.7167, -47.7932)
  arc A429 (16.2167, -48.2932) -> (15.7167, -47.7932) centre (15.7167, -48.2932) ccw
  line L434 (16.2167, -48.2932) -> (16.2167, -61.2932)
  line L435 (58.5792, -9.4057) -> (45.5792, -9.4057)
  arc A430 (45.0792, -8.9057) -> (45.5792, -9.4057) centre (45.5792, -8.9057) ccw
  line L436 (45.0792, -8.9057) -> (45.0792, 4.0943)
  arc A431 (45.5792, 4.5943) -> (45.0792, 4.0943) centre (45.5792, 4.0943) ccw
  line L437 (45.5792, 4.5943) -> (58.5792, 4.5943)
  arc A432 (59.0792, 4.0943) -> (58.5792, 4.5943) centre (58.5793, 4.0943) ccw
  line L438 (59.0792, 4.0943) -> (59.0793, -8.9057)
  arc A433 (58.5792, -9.4057) -> (59.0793, -8.9057) centre (58.5792, -8.9057) ccw
  line L439 (21.7667, -43.0307) -> (34.7667, -43.0307)
  arc A434 (35.2667, -43.5307) -> (34.7667, -43.0307) centre (34.7667, -43.5307) ccw
  line L440 (35.2667, -43.5307) -> (35.2667, -56.5307)
  arc A435 (34.7667, -57.0307) -> (35.2667, -56.5307) centre (34.7667, -56.5307) ccw
  line L441 (34.7667, -57.0307) -> (21.7667, -57.0307)
  arc A436 (21.2667, -56.5307) -> (21.7667, -57.0307) centre (21.7667, -56.5307) ccw
  line L442 (21.2667, -56.5307) -> (21.2667, -43.5307)
  arc A437 (21.7667, -43.0307) -> (21.2667, -43.5307) centre (21.7667, -43.5307) ccw
  line L443 (2.7167, 126.038) -> (15.7167, 126.038)
  arc A438 (16.2168, 125.538) -> (15.7167, 126.038) centre (15.7167, 125.538) ccw
  line L444 (16.2168, 125.538) -> (16.2167, 112.538)
  arc A439 (15.7167, 112.038) -> (16.2167, 112.538) centre (15.7167, 112.538) ccw
  line L445 (15.7167, 112.038) -> (2.7167, 112.038)
  arc A440 (2.2167, 112.538) -> (2.7167, 112.038) centre (2.7167, 112.538) ccw
  line L446 (2.2167, 112.538) -> (2.2167, 125.538)
  arc A441 (2.7167, 126.038) -> (2.2167, 125.538) centre (2.7167, 125.538) ccw
  line L447 (16.2168, 213.6443) -> (16.2168, 200.6443)
  arc A442 (15.7167, 200.1443) -> (16.2168, 200.6443) centre (15.7168, 200.6443) ccw
  line L448 (15.7167, 200.1443) -> (2.7168, 200.1443)
  arc A443 (2.2167, 200.6443) -> (2.7168, 200.1443) centre (2.7168, 200.6443) ccw
  line L449 (2.2167, 200.6443) -> (2.2168, 213.6443)
  arc A444 (2.7168, 214.1443) -> (2.2168, 213.6443) centre (2.7168, 213.6443) ccw
  line L450 (2.7168, 214.1443) -> (15.7168, 214.1443)
  arc A445 (16.2168, 213.6443) -> (15.7168, 214.1443) centre (15.7167, 213.6443) ccw
  arc A446 (-35.8833, -56.5307) -> (-35.3833, -57.0307) centre (-35.3833, -56.5307) ccw
  line L451 (-35.8833, -56.5307) -> (-35.8833, -43.5307)
  arc A447 (-35.3833, -43.0307) -> (-35.8833, -43.5307) centre (-35.3833, -43.5307) ccw
  line L452 (-35.3833, -43.0307) -> (-22.3833, -43.0307)
  arc A448 (-21.8833, -43.5307) -> (-22.3833, -43.0307) centre (-22.3833, -43.5307) ccw
  line L453 (-21.8833, -43.5307) -> (-21.8833, -56.5307)
  arc A449 (-22.3833, -57.0307) -> (-21.8833, -56.5307) centre (-22.3833, -56.5307) ccw
  line L454 (-22.3833, -57.0307) -> (-35.3833, -57.0307)
  line L455 (-6.8083, 156.9943) -> (6.1917, 156.9943)
  arc A450 (6.6917, 156.4943) -> (6.1917, 156.9943) centre (6.1918, 156.4943) ccw
  line L456 (6.6917, 156.4943) -> (6.6917, 143.4943)
  arc A451 (6.1917, 142.9943) -> (6.6917, 143.4943) centre (6.1917, 143.4943) ccw
  line L457 (6.1917, 142.9943) -> (-6.8083, 142.9943)
  arc A452 (-7.3082, 143.4943) -> (-6.8083, 142.9943) centre (-6.8083, 143.4943) ccw
  line L458 (-7.3082, 143.4943) -> (-7.3082, 156.4943)
  arc A453 (-6.8083, 156.9943) -> (-7.3083, 156.4943) centre (-6.8083, 156.4943) ccw
  line L459 (12.2417, -162.0932) -> (25.2417, -162.0932)
  arc A454 (25.7417, -162.5932) -> (25.2417, -162.0932) centre (25.2417, -162.5932) ccw
  line L460 (25.7417, -162.5932) -> (25.7417, -175.5932)
  arc A455 (25.2417, -176.0932) -> (25.7417, -175.5932) centre (25.2417, -175.5932) ccw
  line L461 (25.2417, -176.0932) -> (12.2417, -176.0932)
  arc A456 (11.7417, -175.5932) -> (12.2417, -176.0932) centre (12.2417, -175.5932) ccw
  line L462 (11.7417, -175.5932) -> (11.7417, -162.5932)
  arc A457 (12.2417, -162.0932) -> (11.7417, -162.5932) centre (12.2417, -162.5932) ccw
  line L463 (67.9431, 166.6443) -> (67.9431, 156.6443) construction
  line L464 (67.9431, 156.6443) -> (36.4431, 156.6443)
  line L465 (36.4431, 156.6443) -> (36.4431, 228.6) construction
  line L466 (36.4431, 228.6) -> (67.9431, 228.6)
  line L467 (67.9431, 228.6) -> (67.9431, 156.6443)
  line L468 (37.7668, 228.6) -> (-61.7708, 228.6)
  circle A458 centre (27.4668, 224.6) radius 1.7
  circle A459 centre (-57.5708, 224.6) radius 1.7
  circle A460 centre (-57.1708, -227.4118) radius 2
  circle A461 centre (63.3431, -227.4) radius 2
  line L469 (53.671, -207.2182) -> (40.6292, -207.2182)
  line L470 (40.6292, -207.2182) -> (40.6292, -194.2182)
  line L471 (40.6292, -194.2182) -> (53.671, -194.2182)
  line L472 (53.671, -194.2182) -> (53.671, -207.2182)
  line L473 (53.671, -185.8182) -> (39.7292, -185.8182)
  line L474 (39.7292, -185.8182) -> (39.7292, -161.0182)
  line L475 (39.7292, -161.0182) -> (53.671, -161.0182)
  line L476 (53.671, -161.0182) -> (53.671, -185.8182)
  line L477 (36.4431, 228.6) -> (21.9431, 228.6)
  line L478 (21.9431, 228.6) -> (21.9431, 218.6)
  line L479 (21.9431, 218.6) -> (36.4431, 218.6)
  line L480 (36.4431, 218.6) -> (36.4431, 228.6) construction
  line L481 (36.4431, 218.6) -> (36.4431, 156.6443)
  line L482 (59.9431, 200.6) -> (39.7668, 200.6)
  line L483 (39.7667, 200.6) -> (39.7667, 167.6443)
  line L484 (39.7667, 167.6443) -> (59.9431, 167.6443)
  line L485 (59.9431, 167.6443) -> (59.9431, 200.6)
  line L486 (67.9431, 187.6024) -> (59.9431, 187.6024)
  line L487 (37.7667, 191.1804) -> (39.7667, 191.1804)
  line L488 (51.6, 228.6) -> (51.6, 200.6) construction
  line L489 (51.2813, 166.6443) -> (51.2813, 167.6443)
  line L490 (37.7667, 202.6) -> (37.7667, 165.6443)
  line L491 (37.7667, 165.6443) -> (61.9431, 165.6443)
  line L492 (61.9431, 165.6443) -> (61.9431, 202.6)
  line L493 (61.9431, 202.6) -> (37.7667, 202.6)
  line L494 (38.7667, 201.6) -> (38.7667, 166.6443)
  line L495 (38.7667, 166.6443) -> (60.9431, 166.6443)
  line L496 (60.9431, 166.6443) -> (60.9431, 201.6)
  line L497 (60.9431, 201.6) -> (38.7668, 201.6)
  line L498 (61.9431, 202.6) -> (37.7668, 202.6)
  line L499 (37.7668, 202.6) -> (37.7668, 220.6)
  line L500 (37.7668, 220.6) -> (61.9431, 220.6)
  line L501 (61.9431, 220.6) -> (61.9431, 202.6)
  line L502 (59.9431, 200.6) -> (39.7668, 200.6)
  line L503 (39.7667, 200.6) -> (39.7667, 219.6)
  line L504 (39.7667, 219.6) -> (59.9431, 219.6)
  line L505 (59.9431, 219.6) -> (59.9431, 200.6)
  line L506 (44.4, 220.6) -> (44.4, 219.6)
  line L507 (43.2668, 219.6) -> (67.9431, 219.6)
  line L508 (67.9431, 219.6) -> (67.9431, 202.6)
  line L509 (67.9431, 202.6) -> (43.2668, 202.6)
  line L510 (43.2668, 202.6) -> (43.2668, 219.6)
  line L511 (60.9431, 201.6) -> (67.9431, 201.6)
  line L512 (61.9431, 220.6) -> (67.9431, 220.6)
  line L513 (41, 218.7407) -> (67.9431, 218.7407)
  line L514 (67.9431, 218.7407) -> (67.9431, 203.6)
  line L515 (67.9431, 203.6) -> (41, 203.6)
  line L516 (41, 203.6) -> (41, 218.7407)
  line L517 (43.2668, 202.6) -> (43.2668, 200.6)
  line L518 (67.9431, 228.6) -> (22.0127, 228.6)
  line L519 (22.0127, 228.6) -> (22.0127, 231.6)
  line L520 (22.0127, 231.6) -> (67.9431, 231.6)
  line L521 (67.9431, 231.6) -> (67.9431, 228.6)
  line L522 (19.7667, -118.4115) -> (33.7667, -118.4115)
  arc A462 (34.2667, -118.9115) -> (33.7667, -118.4115) centre (33.7667, -118.9115) ccw
  line L523 (34.2667, -118.9115) -> (34.2667, -124.9115)
  arc A463 (33.7667, -125.4115) -> (34.2667, -124.9115) centre (33.7667, -124.9115) ccw
  line L524 (33.7667, -125.4115) -> (19.7667, -125.4115)
  arc A464 (19.2667, -124.9115) -> (19.7667, -125.4115) centre (19.7667, -124.9115) ccw
  line L525 (19.2667, -124.9115) -> (19.2667, -118.9115)
  arc A465 (19.7667, -118.4115) -> (19.2667, -118.9115) centre (19.7667, -118.9115) ccw
  line L526 (19.7667, -142.2875) -> (33.7667, -142.2875)
  arc A466 (34.2667, -142.7875) -> (33.7667, -142.2875) centre (33.7667, -142.7875) ccw
  line L527 (34.2667, -142.7875) -> (34.2667, -148.7875)
  arc A467 (33.7667, -149.2875) -> (34.2667, -148.7875) centre (33.7667, -148.7875) ccw
  line L528 (33.7667, -149.2875) -> (19.7667, -149.2875)
  arc A468 (19.2667, -148.7875) -> (19.7667, -149.2875) centre (19.7667, -148.7875) ccw
  line L529 (19.2667, -148.7875) -> (19.2667, -142.7875)
  arc A469 (19.7667, -142.2875) -> (19.2667, -142.7875) centre (19.7667, -142.7875) ccw
  dimension "d19" = 10
  dimension "d20" = 31.5
  dimension "d45" = 14.5
  dimension "d46" = 10
  dimension "d47" = 8
  dimension "d48" = 2
  dimension "d49" = 28
  dimension "d50" = 1
  dimension "d53" = 2
  dimension "d58" = 1
  dimension "d64" = 18
  dimension "d65" = 1
  dimension "d68" = 3.5
  dimension "d71" = 1
  dimension "d72" = 0.8593
  dimension "d73" = 1.2332
  dimension "d99" = 3
  constraint coincident L212.start L218.end
  constraint perpendicular L212 L463
  constraint horizontal L464
  constraint vertical L465
  constraint horizontal L466
  constraint vertical L467
  constraint coincident L466 L213.end
  constraint horizontal L477
  constraint vertical L478
  constraint horizontal L479
  constraint vertical L480
  constraint horizontal L482
  constraint vertical L483
  constraint horizontal L484
  constraint vertical L485
  constraint coincident L467 L486.start
  constraint perpendicular L485 L486
  constraint coincident L213 L487.start
  constraint perpendicular L213 L487
  constraint coincident L466 L488.start
  constraint perpendicular L466 L488
  constraint coincident L212 L489.start
  constraint perpendicular L212 L489
  constraint coincident L484 L489.end
  constraint coincident L485 L486.end
  constraint coincident L483 L487.end
  constraint coincident L482 L488.end
  constraint horizontal L498
  constraint vertical L499
  constraint horizontal L500
  constraint vertical L501
  constraint horizontal L502
  constraint vertical L503
  constraint horizontal L504
  constraint vertical L505
  constraint coincident L500 L506.start
  constraint perpendicular L500 L506
  constraint coincident L504 L506.end
  constraint coincident L483.start L503
  constraint horizontal L507
  constraint vertical L508
  constraint horizontal L509
  constraint vertical L510
  constraint coincident L493 L508.end
  constraint coincident L504 L507.start
  constraint coincident L466.end L508
  constraint coincident L467 L511.end
  constraint perpendicular L467 L511
  constraint coincident L467 L512.end
  constraint perpendicular L467 L512
  constraint horizontal L513
  constraint vertical L514
  constraint horizontal L515
  constraint vertical L516
  constraint coincident L508 L514.end
  constraint coincident L502 L517.end
  constraint perpendicular L502 L517
  constraint horizontal L518
  constraint vertical L519
  constraint horizontal L520
  constraint vertical L521
  measures "d19" distance of L212.start L463.end
  measures "d20" distance of L463.end L464.end
  measures "d45" distance of L465.end L477.end
  measures "d46" distance of L465.end L479.end
  measures "d47" distance of L486.start L486.end
  measures "d48" distance of L487.start L487.end
  measures "d49" distance of L488.start L488.end
  measures "d50" distance of L489.start L489.end
  measures "d64" distance of L492.end L500.end
  measures "d65" distance of L506.start L506.end
  measures "d68" distance of L503 L510
  measures "d71" distance of L509 L515
  measures "d72" distance of L504 L513
  measures "d73" distance of L503 L516
  measures "d99" distance of L466.end L520.end